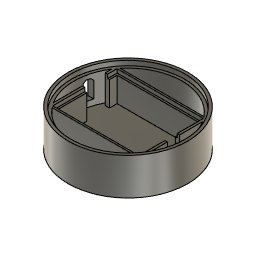
led-lamp-base (Autodesk Fusion 360 design; units mm, degrees)
Autodesk Fusion 360 part; units mm, degrees
sketch "Sketch1" plane through (0, 0, 0) normal (0, 0, 1) x (1, 0, 0)
  circle A0 centre (0, 0) radius 60
  dimension "d1" = 120
  constraint coincident A0.centre origin
  measures "d1" diameter of A0
extrude "Extrude1" add sketch "Sketch1" along normal blind 4 makes body 1
sketch "Sketch2" plane through (0, 0, 0) normal (0, 0, -1) x (1, 0, 0)
  circle A0 centre (0, 0) radius 60
  circle A1 centre (0, 0) radius 63
  dimension "d4" = 3
  constraint coincident A0.centre A1.centre
  measures "d4" distance of A0 A1
extrude "Extrude2" add sketch "Sketch2" against normal blind 39 separate body makes body 2
sketch "Sketch9" plane through (0, 0, 4) normal (0, 0, 1) x (-1, 0, 0)
  circle A0 centre (0, 0) radius 60
  circle A1 centre (0, 0) radius 57
  dimension "d38" = 3
  constraint coincident A0.centre A1.centre
  measures "d38" distance of A0 A1
extrude "Extrude9" add sketch "Sketch9" along normal blind 30 bodies 1 2
sketch "Sketch3" plane through (0, 0, 4) normal (0, 0, 1) x (-1, 0, 0)
  line L0 (43.5, -32) -> (-43.5, -32)
  line L1 (-43.5, -32) -> (-43.5, 32)
  line L2 (-43.5, 32) -> (43.5, 32)
  line L3 (43.5, 32) -> (43.5, -32)
  line L4 (0, 0) -> (43.5, 0)
  line L5 (0, 0) -> (0, -32)
  line L6 (48.0536, -35.9284) -> (-48.0536, -35.9284)
  line L7 (-48.0536, -35.9284) -> (-48.0536, 35.9284)
  line L8 (-48.0536, 35.9284) -> (48.0536, 35.9284)
  line L9 (48.0536, 35.9284) -> (48.0536, -35.9284)
  line L10 (0, -32) -> (0, -35.9284)
  line L11 (-43.5, 0) -> (-48.0536, 0)
  circle A0 centre (0, 0) radius 57
  dimension "d7" = 64
  dimension "d8" = 87
  constraint horizontal L0
  constraint vertical L1
  constraint horizontal L2
  constraint vertical L3
  constraint coincident L4.start L5.start
  constraint midpoint L3 L4.end
  constraint midpoint L0 L5.end
  constraint perpendicular L3 L4
  constraint perpendicular L0 L5
  constraint horizontal L6
  constraint vertical L7
  constraint horizontal L8
  constraint vertical L9
  constraint midpoint L6 L10.end
  constraint collinear L5 L10
  constraint midpoint L1 L11.start
  constraint midpoint L7 L11.end
  constraint collinear L4 L11
  measures "d7" distance of L0.end L1.end
  measures "d8" distance of L0.start L0.end
extrude "Extrude3" add sketch "Sketch3" along normal blind 30 contours L0 L1 L2 L3 L6 L7 L8 L9 L10 L11 A0 | L0 L1 L6 L7 L10 L11 A0 | L6 L9 A0 | L6 L7 A0 | L7 L8 A0 | L8 L9 A0 bodies 1
sketch "Sketch4" plane through (0, 0, 34) normal (0, 0, 1) x (-1, 0, 0)
  line L0 (-43.5, 32) -> (43.5, 32)
  line L1 (43.5, 32) -> (43.5, -32)
  line L2 (43.5, -32) -> (-43.5, -32)
  line L3 (-43.5, -32) -> (-43.5, 32)
  line L4 (44.251, 35.9284) -> (-44.251, 35.9284)
  line L5 (-48.0536, 30.6569) -> (-48.0536, -30.6569)
  line L6 (-44.251, -35.9284) -> (44.251, -35.9284)
  line L7 (48.0536, -30.6569) -> (48.0536, 30.6569)
  line L8 (45.5, -34) -> (-45.5, -34)
  line L9 (-45.5, -34) -> (-45.5, 34)
  line L10 (-45.5, 34) -> (45.5, 34)
  line L11 (45.5, 34) -> (45.5, -34)
  line L12 (48.0536, 0) -> (45.5, 0)
  line L13 (0, -32) -> (0, -34)
  arc A0 (-48.0536, 30.6569) -> (-48.0536, -30.6569) centre (0, 0) ccw
  arc A1 (-44.251, -35.9284) -> (44.251, -35.9284) centre (0, 0) ccw
  arc A2 (44.251, 35.9284) -> (-44.251, 35.9284) centre (0, 0) ccw
  circle A3 centre (0, 0) radius 60
  arc A4 (48.0536, -30.6569) -> (48.0536, 30.6569) centre (0, 0) ccw
  dimension "d11" = 2
  dimension "d12" = 2
  constraint horizontal L8
  constraint vertical L9
  constraint horizontal L10
  constraint vertical L11
  constraint midpoint L7 L12.start
  constraint midpoint L11 L12.end
  constraint perpendicular L11 L12
  constraint midpoint L2 L13.start
  constraint midpoint L8 L13.end
  constraint perpendicular L8 L13
  measures "d11" distance of L2 L8
  measures "d12" distance of L3 L9
extrude "Extrude4" cut sketch "Sketch4" against normal blind 4 contours L8 L9 L10 L11 bodies 1
sketch "Sketch5" plane through (0, 0, 34) normal (0, 0, 1) x (-1, 0, 0)
  line L0 (-45.5, -34) -> (-45.5, 34)
  line L1 (-45.5, 34) -> (45.5, 34)
  line L2 (45.5, 34) -> (45.5, -34)
  line L3 (45.5, -34) -> (-45.5, -34)
  line L4 (44.251, 35.9284) -> (-44.251, 35.9284)
  line L5 (-48.0536, 30.6569) -> (-48.0536, -30.6569)
  line L6 (-44.251, -35.9284) -> (44.251, -35.9284)
  line L7 (48.0536, -30.6569) -> (48.0536, 30.6569)
  line L8 (48.0536, -24) -> (43.5, -24)
  line L9 (43.5, -24) -> (43.5, 0)
  line L10 (43.5, 0) -> (48.0536, 0)
  line L11 (48.0536, 0) -> (48.0536, -24)
  line L12 (-43.5, -32) -> (43.5, -32)
  line L13 (43.5, -32) -> (43.5, 32)
  arc A0 (-48.0536, 30.6569) -> (-48.0536, -30.6569) centre (0, 0) ccw
  arc A1 (-44.251, -35.9284) -> (44.251, -35.9284) centre (0, 0) ccw
  arc A2 (44.251, 35.9284) -> (-44.251, 35.9284) centre (0, 0) ccw
  circle A3 centre (0, 0) radius 60
  arc A4 (48.0536, -30.6569) -> (48.0536, 30.6569) centre (0, 0) ccw
  dimension "d15" = 8
  dimension "d16" = 32
  constraint horizontal L8
  constraint vertical L9
  constraint horizontal L10
  constraint vertical L11
  constraint collinear L7 L11
  constraint collinear L9 L13
  measures "d15" distance of L8 L12
  measures "d16" distance of L10 L12
extrude "Extrude5" cut sketch "Sketch5" against normal up to surface (30 mm away) contours L2 L8 L9 L10 L13 | L2 L7 L8 L10 L11 bodies 1
sketch "Sketch6" plane through (0, 0, 34) normal (0, 0, 1) x (-1, 0, 0)
  line L0 (45.5, 0) -> (48.0536, 0)
  line L1 (48.0536, 0) -> (48.0536, 30.6569)
  line L2 (44.251, 35.9284) -> (-44.251, 35.9284)
  line L3 (-48.0536, 30.6569) -> (-48.0536, -30.6569)
  line L4 (-44.251, -35.9284) -> (44.251, -35.9284)
  line L5 (48.0536, -24) -> (45.5, -24)
  line L6 (45.5, -24) -> (45.5, -34)
  line L7 (45.5, -34) -> (-45.5, -34)
  line L8 (-45.5, -34) -> (-45.5, 34)
  line L9 (-45.5, 34) -> (45.5, 34)
  line L10 (-43.5, -6.5) -> (-48.0536, -6.5)
  line L11 (-48.0536, -6.5) -> (-48.0536, 6.5)
  line L12 (-48.0536, 6.5) -> (-43.5, 6.5)
  line L13 (-43.5, 6.5) -> (-43.5, -6.5)
  line L14 (-43.5, 32) -> (-43.5, -32)
  line L15 (0, 0) -> (-43.5, 0)
  arc A0 (48.0536, -30.6569) -> (48.0536, 30.6569) centre (0, 0) ccw
  line L16 (48.0536, -30.6569) -> (48.0536, -24)
  line L17 (45.5, 34) -> (45.5, 0)
  arc A1 (-48.0536, 30.6569) -> (-48.0536, -30.6569) centre (0, 0) ccw
  arc A2 (-44.251, -35.9284) -> (44.251, -35.9284) centre (0, 0) ccw
  arc A3 (44.251, 35.9284) -> (-44.251, 35.9284) centre (0, 0) ccw
  circle A4 centre (0, 0) radius 60
  dimension "d19" = 13
  constraint horizontal L10
  constraint vertical L11
  constraint horizontal L12
  constraint vertical L13
  constraint collinear L3 L11
  constraint collinear L13 L14
  constraint coincident L15.start A0.centre
  constraint midpoint L13 L15.end
  constraint perpendicular L13 L15
  measures "d19" distance of L10.end L11.end
extrude "Extrude6" cut sketch "Sketch6" against normal up to surface (30 mm away) contours L8 L10 L12 L13 L14 | L3 L8 L10 L11 L12 bodies 1
ref_plane "WorkPlane1" through (-100, 0, 0) normal (1, 0, 0) x (0, 1, 0)
sketch "Sketch8" plane through (-100, 0, 0) normal (1, 0, 0) x (0, 1, 0)
  line L0 (18, 27) -> (9, 27)
  line L1 (9, 27) -> (9, 10)
  line L2 (9, 10) -> (18, 10)
  line L3 (18, 10) -> (18, 27)
  line L4 (18, 27) -> (15.5, 29.5)
  line L5 (15.5, 29.5) -> (11.5, 29.5)
  line L6 (11.5, 29.5) -> (9, 27)
  dimension "d29" = 10
  dimension "d30" = 9
  dimension "d31" = 17
  dimension "d32" = 9
  dimension "d35" = 45
  dimension "d36" = 45
  dimension "d37" = 4
  constraint horizontal L0
  constraint vertical L1
  constraint horizontal L2
  constraint vertical L3
  constraint perpendicular L3 L5
  measures "d29" distance of origin L2
  measures "d30" distance of origin L1
  measures "d31" distance of L0.start L2.end
  measures "d32" distance of L0.start L0.end
  measures "d35" angle of L0 L6
  measures "d36" angle of L0 L4
  measures "d37" distance of L4.end L5.end
extrude "Extrude8" cut sketch "Sketch8" along normal up to surface end surface at (-50.7358, -25.9784, 24) on bodies 1 bodies 1
